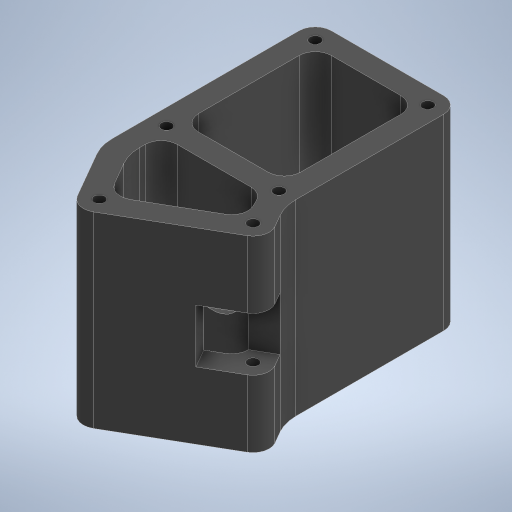
# Autodesk Inventor part: leg_upper_middle
Saved by Autodesk Inventor 2024.1 (Build 281209000, 209)
## iProperties
Created: 2024-02-11
Part Number: leg_upper_middle
Material: 一般
Document SubType Name: Modeling
Designer: hibik
Density: 1 g/cm^3
Appearance: 既定
Author: hibik
Autodesk Inventor part; units mm, degrees
ref_plane "YZ Plane" through (0, 0, 0) normal (1, 0, 0) x (0, 1, 0)
ref_plane "XZ Plane" through (0, 0, 0) normal (0, 1, 0) x (-1, 0, 0)
ref_plane "XY Plane" through (0, 0, 0) normal (0, 0, 1) x (1, 0, 0)
sketch "スケッチ1" plane through (0, 0, 0) normal (0, 1, 0) x (-1, 0, 0)
  line L0 (0, 0) -> (4, 0)
  line L1 (4, 0) -> (4, -40)
  line L2 (4, -40) -> (0, -40)
  line L3 (0, -40) -> (0, 0)
  line L4 (-3.5, 12.9904) -> (-6.9641, 10.9904)
  line L5 (-6.9641, 10.9904) -> (0.5359, -2)
  line L6 (0.5359, -2) -> (4, 0)
  line L7 (4, 0) -> (-3.5, 12.9904)
  line L8 (4, -40) -> (-23, -40)
  line L9 (-23, -40) -> (-23, -36)
  line L10 (-23, -36) -> (4, -36)
  line L11 (4, -36) -> (4, -40)
  line L12 (-3.5, 12.9904) -> (-1.5, 9.5263)
  line L13 (-1.5, 9.5263) -> (-24.8827, -3.9737)
  line L14 (-24.8827, -3.9737) -> (-26.8827, -0.5096)
  line L15 (-26.8827, -0.5096) -> (-3.5, 12.9904)
  line L16 (-23, -40) -> (-19, -40)
  line L17 (-19, -40) -> (-19, -7.2346)
  line L18 (-19, -7.2346) -> (-23, -7.2346)
  line L19 (-23, -7.2346) -> (-23, -40)
  line L20 (-26.8827, -0.5096) -> (-23.4186, 1.4904)
  line L21 (-23.4186, 1.4904) -> (-19.5359, -5.2346)
  line L22 (-19.5359, -5.2346) -> (-23, -7.2346)
  line L23 (-23, -7.2346) -> (-26.8827, -0.5096)
  line L24 (-23, -7.2346) -> (4, -7.2346)
  line L25 (4, -7.2346) -> (4, -11.2346)
  line L26 (4, -11.2346) -> (-23, -11.2346)
  line L27 (-23, -11.2346) -> (-23, -7.2346)
  line L28 (-19.5359, -5.2346) -> (-19, -7.2346)
  point P0 (0, -1.0718)
  point P1 (-21.4186, -1.9737)
  point P2 (-4.9641, 7.5263)
  point P3 (-24.8827, -3.9737)
  point P4 (0, -36)
  point P5 (-19, -36)
  point P6 (-19, -11.2346)
  point P7 (0, -11.2346)
  point P8 (0, -7.2346)
  dimension "d2" = 4
  dimension "d3" = 30
  dimension "d5" = 40
  dimension "d6" = 15
  dimension "d7" = 27
  dimension "d8" = 27
  constraints: 58 end point, 14 parallel, 7 perpendicular, 6 equal length, 4 horizontal, 3 point on line
  measures "d2" distance of L1.end L2.end
  measures "d3" angle of L1 L7
  measures "d5" distance of L0.end L1.end
  measures "d6" distance between parallel lines of L6 L4
  measures "d7" distance of L1.end L8.end
  measures "d8" distance between parallel lines of L7 L14
extrude "押し出し1" add sketch "スケッチ1" along normal blind 35 contours L3 L5 L13 L7 L0 | L0 L6 L5 L3 | L1 L24 L3 L5 L6 | L1 L26 L3 L24 | L13 L5 L4 L7 | L3 L26 L17 L24 | L13 L21 L15 L5 | L1 L10 L3 L26 | L17 L26 L19 L18 | L18 L22 L28 | L21 L22 L23 L13 | L13 L14 L15 L21 | L1 L2 L3 L10 | L3 L8 L17 L10 | L17 L10 L19 L26 | L17 L8 L9 L10
fillet "フィレット1" radius 8 4 edges at (-4, 17.5, 0) (23, 17.5, -7.2346) (19.5359, 17.5, -5.2346) (0, 17.5, -1.0718)
fillet "フィレット2" radius 3 12 edges at (3.5, 17.5, 12.9904) (26.8827, 17.5, -0.5096) (23, 17.5, -40) (-4, 17.5, -40) (0, 17.5, -11.2346) (19, 17.5, -36) (0, 17.5, -36) (19, 17.5, -11.2346) (4.9641, 17.5, 7.5263) (0, 17.5, -7.2346) (19, 17.5, -7.2346) (21.4186, 17.5, -1.9737)
sketch "スケッチ2" plane through (0, 35, 0) normal (0, 1, 0) x (1, 0, 0)
  circle A0 centre (4.5981, -8.8923) radius 1
  arc A1 (2, -10.3923) -> (6.0981, -11.4904) centre (4.5981, -8.8923) ccw projected
  circle A2 centre (22.7846, 1.6077) radius 1
  circle A3 centre (20, 37) radius 1
  circle A4 centre (20, 9.2346) radius 1
  circle A5 centre (-1, 9.2346) radius 1
  circle A6 centre (-1, 37) radius 1
  arc A7 (24.2846, -0.9904) -> (25.3827, 3.1077) centre (22.7846, 1.6077) ccw projected
  arc A8 (-1, 40) -> (-4, 37) centre (-1, 37) ccw projected
  arc A9 (23, 37) -> (20, 40) centre (20, 37) ccw projected
  line L0 (3, 7.2346) -> (16.7785, 7.2346) projected
  line L1 (16, 11.2346) -> (3, 11.2346) projected
  point P0 (0, 0)
  dimension "d10" = 2
  dimension "d11" = 2
  dimension "d12" = 2
  dimension "d13" = 2
  dimension "d14" = 2
  dimension "d15" = 2
  dimension "d16" = 2
  dimension "d17" = 2
  constraints: 6 centre point, 4 concentric, 2 vertical alignment, 1 horizontal alignment
  measures "d10" diameter of A0
  measures "d11" diameter of A2
  measures "d12" diameter of A3
  measures "d13" diameter of A4
  measures "d14" diameter of A5
  measures "d15" diameter of A6
  measures "d16" distance from line of A5.centre L0
  measures "d17" distance from line of A5.centre L1
extrude "押し出し2" cut sketch "スケッチ2" against normal through all
sketch "スケッチ3" plane through (24.0718, 0, -5.3782) normal (0.8660254, 0, -0.5) x (-0.5, 0, -0.8660254)
  line L0 (-2.6218, 0) -> (-2.6218, 35) projected
  line L1 (-2.6218, 0) -> (0, 0) projected
  line L2 (0, 35) -> (0, 0) projected
  line L3 (-2.6218, 35) -> (0, 35) projected
  line L4 (0, 12.5) -> (-14.5476, 12.5)
  line L5 (-14.5476, 12.5) -> (-14.5476, 22.5)
  line L6 (-14.5476, 22.5) -> (0, 22.5)
  line L7 (0, 22.5) -> (0, 12.5)
  line L8 (0, 35) -> (0, 0) projected
  point P0 (7.3782, 0)
  point P1 (0, 17.5)
  point P2 (0, 17.5)
  dimension "d20" = 10
  constraints: 8 end point, 2 midpoint, 2 parallel, 1 coincident, 1 horizontal, 1 perpendicular, 1 point on line
  measures "d20" distance of L4.end L5.end
extrude "押し出し3" cut sketch "スケッチ3" against normal blind 10 contours L4 L5 L6 L0 | L0 L6 L2 L4
sketch "スケッチ5" plane through (16, 0, -11.2346) normal (0, 0, -1) x (-1, 0, 0)
  line L0 (0, 0) -> (0, 35) projected
  line L1 (0, 0) -> (13, 0) projected
  line L2 (13, 35) -> (13, 0) projected
  line L3 (0, 35) -> (13, 35) projected
  line L4 (0, 35) -> (13, 35) projected
  line L5 (13, 35) -> (0, 0)
  line L6 (13, 0) -> (0, 35)
  circle A0 centre (6.5, 17.5) radius 6
  point P0 (16, 0)
  dimension "d26" = 12
  constraints: 4 end point, 1 centre point, 1 midpoint
  measures "d26" diameter of A0
extrude "押し出し5" cut sketch "スケッチ5" against normal up to surface (4 mm away) contours A0 L6 L5 | L5 L6 A0 | A0 L5 L6 | L6 L5 A0
equation "\"d16\" = d17"
